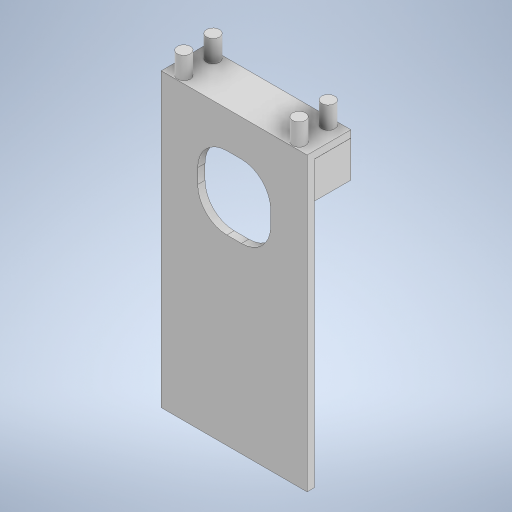
# Autodesk Inventor part: fixation_v02
Saved by Autodesk Inventor 2023 (Build 270158000, 158)
## iProperties
Created: 2021-04-13
Part Number: fixation_v02
Material: Generic
Document SubType Name: Modeling
Designer: KAMPFF-LAB-BEHAVIOR
Density: 1 g/cm^3
Appearance: Default
Author: KAMPFF-LAB-BEHAVIOR
Autodesk Inventor part; units mm, degrees
ref_plane "YZ Plane" through (0, 0, 0) normal (1, 0, 0) x (0, 1, 0)
ref_plane "XZ Plane" through (0, 0, 0) normal (0, 1, 0) x (-1, 0, 0)
ref_plane "XY Plane" through (0, 0, 0) normal (0, 0, 1) x (1, 0, 0)
sketch "Sketch1" plane through (0, 0, 0) normal (0, 0, 1) x (1, 0, 0)
  line L0 (-50, -100) -> (50, -100)
  line L1 (50, -100) -> (50, 100)
  line L2 (50, 100) -> (-50, 100)
  line L3 (-50, 100) -> (-50, -100)
  line L4 (-50, -100) -> (50, 100) construction
  line L5 (50, -100) -> (-50, 100) construction
  point P0 (0, 0)
  dimension "d0" = 100
  dimension "d1" = 200
  constraints: 12 end point, 2 midpoint, 2 parallel, 1 horizontal, 1 perpendicular
  measures "d0" distance of L2.end L1.end
  measures "d1" distance of L1.end L0.end
extrude "Extrusion1" add sketch "Sketch1" along normal blind 5
sketch "Sketch6" plane through (0, 0, 5) normal (0, 0, 1) x (1, 0, 0)
  line L0 (4.9986, 75) -> (-5.0014, 75)
  line L1 (-25.0014, 55) -> (-25.0014, 45)
  line L2 (-5.0014, 25) -> (4.9986, 25)
  line L3 (24.9986, 45) -> (24.9986, 55)
  line L4 (24.9986, 75) -> (-25.0014, 25) construction
  line L5 (-25.0014, 75) -> (24.9986, 25) construction
  arc A0 (4.9986, 25) -> (24.9986, 45) centre (4.9986, 45) ccw
  arc A1 (24.9986, 55) -> (4.9986, 75) centre (4.9986, 55) ccw
  arc A2 (-5.0014, 75) -> (-25.0014, 55) centre (-5.0014, 55) ccw
  arc A3 (-25.0014, 45) -> (-5.0014, 25) centre (-5.0014, 45) ccw
  point P0 (0, 0)
  point P1 (-0.0014, 50)
  dimension "d21" = 50
  dimension "d22" = 50
  dimension "d23" = 20
  constraints: 12 end point, 8 point on circle, 8 point on line, 8 tangent, 4 centre point, 3 equal radius, 2 midpoint, 2 parallel, 1 horizontal, 1 perpendicular
  measures "d21" distance of L5.end L4.end
  measures "d22" distance of L4.end L5.start
  measures "d23" radius of A0
extrude "Extrusion6" cut sketch "Sketch6" against normal blind 5
sketch "Sketch15" plane through (-50, 100, 5) normal (0, 1, 0) x (1, 0, 0)
  line L0 (100, 0) -> (0, 0) projected
  line L1 (0, 0) -> (100, 0)
  line L2 (100, 0) -> (100, 30)
  line L3 (100, 30) -> (0, 30)
  line L4 (0, 30) -> (0, 0)
  point P0 (50, 5)
  dimension "d46" = 100
  dimension "d47" = 30
  constraints: 8 end point, 2 parallel, 1 horizontal, 1 perpendicular
  measures "d46" distance of L3.end L2.end
  measures "d47" distance of L2.end L1.end
sketch "Sketch16" plane through (-50, 100, 5) normal (0, 1, 0) x (1, 0, 0)
  circle A0 centre (10.5, 5) radius 4.5
  circle A1 centre (89.5, 5) radius 4.5
  circle A2 centre (10.5, 25) radius 4.5
  circle A3 centre (89.5, 25) radius 4.5
  point P0 (50, 5)
  dimension "d48" = 9
  dimension "d49" = 9
  dimension "d50" = 9
  dimension "d51" = 9
  constraints: 4 centre point
  measures "d48" diameter of A0
  measures "d49" diameter of A1
  measures "d50" diameter of A2
  measures "d51" diameter of A3
extrude "Extrusion11" add sketch "Sketch15" against normal blind 5
extrude "Extrusion12" add sketch "Sketch16" along normal blind 15
sketch "Sketch17" plane through (50, 100, -25) normal (0, 0, -1) x (-1, 0, 0)
  line L0 (100.0829, 0) -> (0.0829, 0)
  line L1 (0.0829, 0) -> (0.0829, -30)
  line L2 (0.0829, -30) -> (100.0829, -30)
  line L3 (100.0829, -30) -> (100.0829, 0)
  point P0 (50, -100)
  dimension "d56" = 100
  dimension "d57" = 30
  constraints: 8 end point, 2 parallel, 1 horizontal, 1 perpendicular
  measures "d56" distance of L2.end L1.end
  measures "d57" distance of L1.end L0.end
extrude "Extrusion13" add sketch "Sketch17" against normal blind 5
sketch "Sketch18" plane through (49.9171, 70, -25) normal (1, 0, 0) x (0, 0, -1)
  line L0 (0, 0) -> (-5, 0) projected
  line L1 (-30, 30) -> (-30, -170) projected
  line L2 (0, 0) -> (-30, 0)
  line L3 (-30, 0) -> (-30, 30)
  line L4 (-30, 30) -> (0, 30)
  line L5 (0, 30) -> (0, 0)
  point P0 (-25, -70)
  constraints: 8 end point, 2 parallel, 1 horizontal, 1 perpendicular
extrude "Extrusion14" add sketch "Sketch18" against normal blind 5
sketch "Sketch20" plane through (-50, -100, 5) normal (-1, 0, 0) x (0, 0, 1)
  line L0 (-30, 200) -> (0, 200) projected
  line L1 (-30, 170) -> (-30, 200) projected
  line L2 (0, 200) -> (-30, 200)
  line L3 (-30, 200) -> (-30, 170)
  line L4 (-30, 170) -> (0, 170)
  line L5 (0, 170) -> (0, 200)
  point P0 (-5, 100)
  constraints: 8 end point, 2 parallel, 1 horizontal, 1 perpendicular
extrude "Extrusion16" add sketch "Sketch20" against normal blind 5
body "Solid1"
